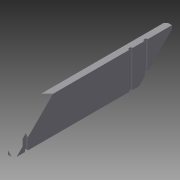
# Autodesk Inventor part: Dish_Front_Base
Saved by Autodesk Inventor 2014 (Build 180170000, 170)
## iProperties
Created: 2015-01-07
Part Number: Dish_Front_Base
Material: Generic
Document SubType Name: Modeling
Designer: Owner
Density: 1 g/cm^3
Appearance: Default
Author: Owner
Autodesk Inventor part; units mm, degrees
ref_plane "YZ Plane" through (0, 0, 0) normal (1, 0, 0) x (0, 1, 0)
ref_plane "XZ Plane" through (0, 0, 0) normal (0, 1, 0) x (-1, 0, 0)
ref_plane "XY Plane" through (0, 0, 0) normal (0, 0, 1) x (1, 0, 0)
sketch "Sketch1" plane through (0, 0, 0) normal (0, 1, 0) x (-1, 0, 0)
  line L0 (39.1686, 2.0724) -> (39.1686, -163.0276)
  line L1 (45.5186, 2.0724) -> (45.5186, -163.0276)
  line L2 (39.1686, -137.6276) -> (40.7561, -137.6276)
  line L3 (40.7561, -137.6276) -> (40.7561, -134.4526)
  line L4 (40.7561, -134.4526) -> (39.1686, -134.4526)
  line L5 (39.1686, -134.4526) -> (39.1686, -137.6276)
  line L6 (39.1686, -163.0276) -> (45.5186, -163.0276)
  line L7 (39.1686, 2.0724) -> (45.5186, 2.0724)
  line L8 (39.1686, -121.7526) -> (40.7561, -121.7526)
  line L9 (40.7561, -121.7526) -> (40.7561, -118.5776)
  line L10 (40.7561, -118.5776) -> (39.1686, -118.5776)
  line L11 (39.1686, -118.5776) -> (39.1686, -121.7526)
  line L12 (39.1686, -9.2306) -> (40.7561, -9.2306)
  line L13 (40.7561, -9.2306) -> (40.7561, -12.4056)
  line L14 (40.7561, -12.4056) -> (39.1686, -12.4056)
  line L15 (39.1686, -12.4056) -> (39.1686, -9.2306)
  point P0 (0, 0)
  dimension "d0" = 6.35
  dimension "d5" = 165.1
  dimension "d10" = 3.175
  dimension "d11" = 1.5875
  dimension "d14" = 3.175
  dimension "d15" = 3.175
  dimension "d17" = 1.5875
  dimension "d18" = 112.522
  dimension "d19" = 12.7
  dimension "d20" = 25.4
  dimension "d21" = 1.5875
  constraints: 32 end point, 6 parallel, 5 perpendicular, 3 horizontal, 3 point on line, 2 vertical
  measures "d0" distance between parallel lines of L1 L0
  measures "d5" distance of L0.start L0.end
  measures "d10" distance of L2.end L3.end
  measures "d11" distance of L3.end L4.end
  measures "d14" distance of L12.end L13.end
  measures "d15" distance of L8.end L9.end
  measures "d17" distance of L13.end L14.end
  measures "d18" distance between parallel lines of L8 L12
  measures "d19" distance between parallel lines of L8 L4
  measures "d20" distance between parallel lines of L6 L2
  measures "d21" distance between parallel lines of L11 L9
extrude "Extrusion1" add sketch "Sketch1" along normal blind 38.1 contours L7 L1 L6 L0 L2 L3 L4 L8 L9 L10 L14 L13 L12
body "Solid1"
